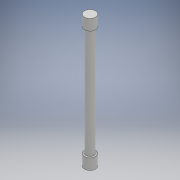
# Autodesk Inventor part: TirasLaterales
Saved by Autodesk Inventor 2017 SP1 (Build 210196100, 196)
## iProperties
Part Number: TirasLaterales
Material: Genérico
Document SubType Name: Modeling
Designer: Juan
Density: 1 g/cm^3
Appearance: Valor por defecto
Author: Juan
Autodesk Inventor part; units mm, degrees
ref_plane "YZ Plane" through (0, 0, 0) normal (1, 0, 0) x (0, 1, 0)
ref_plane "XZ Plane" through (0, 0, 0) normal (0, 1, 0) x (-1, 0, 0)
ref_plane "XY Plane" through (0, 0, 0) normal (0, 0, 1) x (1, 0, 0)
sketch "Boceto1" plane through (0, 0, 0) normal (1, 0, 0) x (0, 1, 0)
  line L0 (0, 0) -> (0, -20)
  line L1 (0, -20) -> (3, -20)
  line L2 (0, 0) -> (10, 0)
  line L3 (3, -20) -> (3, -120)
  line L4 (0, -240) -> (0, -220)
  line L5 (0, -220) -> (3, -220)
  line L6 (0, -240) -> (10, -240)
  line L7 (3, -220) -> (3, -120)
  line L8 (10, 0) -> (10, -240)
  dimension "d1" = 20
  dimension "d2" = 3
  dimension "d3" = 10
  dimension "d4" = 100
  dimension "d11" = 100
  dimension "d12" = 240
  constraints: 18 end point, 4 vertical, 3 parallel, 1 coincident, 1 horizontal, 1 perpendicular
  measures "d1" distance of L0.start L0.end
  measures "d2" distance of L0.end L1.end
  measures "d3" distance of L0.start L2.end
  measures "d4" distance of L1.end L3.end
  measures "d11" distance of L7.start L3.end
  measures "d12" distance of L2.end L6.end
revolve "Revolución1" add sketch "Boceto1" angle 360 about axis through (0, 10, 0) along (0, 0, -1)
equation "\"d11\" = d4"
